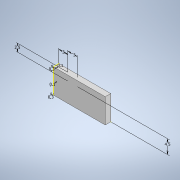
# Autodesk Inventor part: bobecase
Saved by Autodesk Inventor 2022 (Build 260153000, 153)
## iProperties
Created: 2021-10-13
Part Number: bobecase
Material: 일반
Document SubType Name: Modeling
Designer: ELEC-01
Density: 1 g/cm^3
Appearance: 기본값
Author: ELEC-01
Autodesk Inventor part; units mm, degrees
ref_plane "YZ Plane" through (0, 0, 0) normal (1, 0, 0) x (0, 1, 0)
ref_plane "XZ Plane" through (0, 0, 0) normal (0, 1, 0) x (-1, 0, 0)
ref_plane "XY Plane" through (0, 0, 0) normal (0, 0, 1) x (1, 0, 0)
sketch "스케치1" plane through (0, 0, 0) normal (0, 0, 1) x (1, 0, 0)
  line L0 (0, 0) -> (17, 0)
  line L1 (17, 0) -> (17, 8)
  line L2 (17, 8) -> (0, 8)
  line L3 (0, 8) -> (0, 0)
  line L4 (0, 4.8) -> (17, 4.8)
  line L5 (15, 8) -> (15, 0)
  dimension "d0" = 17
  dimension "d1" = 8
  dimension "d3" = 4.8
  dimension "d4" = 15
  constraints: 12 end point, 4 point on line, 3 perpendicular, 2 parallel, 1 horizontal
  measures "d0" distance of L2.end L1.end
  measures "d1" distance of L1.end L0.end
  measures "d3" distance between parallel lines of L0 L4
  measures "d4" distance between parallel lines of L3 L5
extrude "돌출1" add sketch "스케치1" along normal mid plane 1.8
sketch "스케치3" plane through (0, 0, 0.9) normal (-1, 0, 0) x (0, 0, 1)
  line L0 (-1.8, 0) -> (0, 0) projected
  line L1 (-1.8, 0) -> (-1.8, 8) projected
  line L2 (-1.7, 7.7) -> (-0.1, 7.7)
  line L3 (-0.1, 7.7) -> (-0.1, 0.3)
  line L4 (-0.1, 0.3) -> (-1.7, 0.3)
  line L5 (-1.7, 0.3) -> (-1.7, 7.7)
  line L6 (-1.8, 8) -> (0, 8) projected
  line L7 (0, 8) -> (0, 0) projected
  point P0 (-0.9, 0)
  dimension "d11" = 0.3
  dimension "d12" = 0.3
  dimension "d13" = 0.1
  dimension "d14" = 0.1
  constraints: 8 end point, 2 parallel, 1 horizontal, 1 perpendicular
  measures "d11" distance between parallel lines of L6 L2
  measures "d12" distance between parallel lines of L0 L4
  measures "d13" distance between parallel lines of L7 L3
  measures "d14" distance between parallel lines of L1 L5
sketch "스케치5" plane through (0, 0, -0.9) normal (0, 0, -1) x (-1, 0, 0)
  line L0 (-6, 7) -> (-3, 7)
  line L1 (-3, 7) -> (-3, 4.5)
  line L2 (-3, 4.5) -> (-6, 4.5)
  line L3 (-6, 4.5) -> (-6, 7)
  line L4 (0, 0) -> (0, 8) projected
  line L5 (-17, 0) -> (0, 0) projected
  dimension "d15" = 3
  dimension "d16" = 2.5
  dimension "d17" = 3
  dimension "d18" = 4.5
  constraints: 8 end point, 2 parallel, 1 horizontal, 1 perpendicular
  measures "d15" distance of L0.start L0.end
  measures "d16" distance of L0.end L1.end
  measures "d17" distance between parallel lines of L4 L1
  measures "d18" distance between parallel lines of L5 L2
